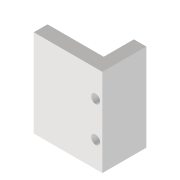
# Autodesk Inventor part: 10_Motormount
Saved by Autodesk Inventor 2022 (Build 260153000, 153)
## iProperties
Created: 2022-04-18
Part Number: 10_Motormount
Material: Generic
Document SubType Name: Modeling
Designer: Prakash Lab
Density: 1 g/cm^3
Appearance: Default
Author: Prakash Lab
Autodesk Inventor part; units mm, degrees
ref_plane "YZ Plane" through (0, 0, 0) normal (1, 0, 0) x (0, 1, 0)
ref_plane "XZ Plane" through (0, 0, 0) normal (0, 1, 0) x (-1, 0, 0)
ref_plane "XY Plane" through (0, 0, 0) normal (0, 0, 1) x (1, 0, 0)
sketch "Sketch1" plane through (0, 0, 0) normal (0, 0, 1) x (1, 0, 0)
  line L0 (2, 10.1) -> (2, 16.1) projected
  line L1 (2, 10.1) -> (2, -23.7) projected
  line L2 (-18.5, 15.1) -> (-18.5, 8.9) projected
  line L3 (-18.5, 8.9) -> (-18.5, -8.9) projected
  line L4 (-18.5, -8.9) -> (-18.5, -15.9) projected
  circle A0 centre (4.0729, 6.3227) radius 1.4 projected
  circle A1 centre (4.0729, -6.5955) radius 1.4 projected
  line L5 (6.5, -92.7) -> (6.5, 10.1) projected
  line L6 (6.5, 8.6074) -> (-18.5, 8.6074)
  line L7 (-18.5, 8.6074) -> (-18.5, -15.9)
  line L8 (-18.5, -15.9) -> (6.5, -15.9)
  line L9 (6.5, -15.9) -> (6.5, 8.6074)
  circle A2 centre (4.0729, 6.3227) radius 1.65
  circle A3 centre (4.0729, -6.5955) radius 1.65
  line L10 (-17, 8.9) -> (0, 8.9) projected
  point P0 (0, 0)
  point P1 (6.5, -15.9)
  point P2 (6.5, 8.6074)
  point P3 (-18.5, 13.8571)
  point P4 (-18.5, 8.6074)
  dimension "d0" = 25
  dimension "d1" = 3.3
  dimension "d2" = 3.3
  constraints: 8 end point, 2 centre point, 2 coincident, 2 parallel, 1 horizontal, 1 perpendicular
  measures "d0" distance of L8.end L4.end
  measures "d1" diameter of A2
  measures "d2" diameter of A3
extrude "Extrusion1" add sketch "Sketch1" along normal blind 5 contours L6 L5 L8 L1 | L1 L8 L4 L3 L6
sketch "Sketch2" plane through (0, 0, 0) normal (0, 0, -1) x (-1, 0, 0)
  line L0 (-6.5, -92.7) -> (-6.5, 27.1) projected
  line L1 (-2, 16.1) -> (-2, -23.7) projected
  line L2 (-6.5, 8.6074) -> (18.5, 8.6074) projected
  line L3 (18.5, -15.9) -> (-6.5, -15.9) projected
  circle A0 centre (-4.0729, -6.5955) radius 1.65 projected
  circle A1 centre (-4.0729, 6.3227) radius 1.65 projected
  line L4 (-6.5, 16.1) -> (-2, 16.1)
  line L5 (-2, 16.1) -> (-2, -15.9)
  line L6 (-2, -15.9) -> (-6.5, -15.9)
  line L7 (-6.5, -15.9) -> (-6.5, 16.1)
  point P0 (0, 0)
  point P1 (18.5, 16.1)
  point P2 (-2, 8.6074)
  constraints: 8 end point, 2 parallel, 2 point on line, 1 horizontal, 1 perpendicular, 1 other
ref_plane "Work Plane1" through (-79, -96.7, -11) normal (0, 0, 1) x (1, 0, 0)
extrude "Extrusion2" add sketch "Sketch2" along normal up to surface (11 mm away) contours L0 L2 L1 L3
body "Solid1"
